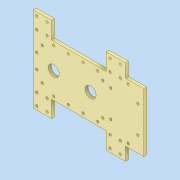
# Autodesk Inventor part: 130底盘5.0
Saved by Autodesk Inventor 2019 (Build 230136000, 136)
## iProperties
Created: 2020-11-07
Part Number: 130底盘5.0
Material: 尼龙 6/6
Document SubType Name: Modeling
Designer: Wang Hua
Density: 1.13 g/cm^3
Appearance: 尼龙 6
Author: Wang Hua
Autodesk Inventor part; units mm, degrees
ref_plane "YZ Plane" through (0, 0, 0) normal (1, 0, 0) x (0, 1, 0)
ref_plane "XZ Plane" through (0, 0, 0) normal (0, 1, 0) x (-1, 0, 0)
ref_plane "XY Plane" through (0, 0, 0) normal (0, 0, 1) x (1, 0, 0)
sketch "草图1" plane through (0, 0, 0) normal (0, 0, 1) x (1, 0, 0)
  line L0 (-136.9893, 0) -> (-136.9893, 58)
  line L1 (-136.9893, 58) -> (-111.9893, 58)
  line L2 (-111.9893, 58) -> (-111.9893, 35)
  line L3 (-111.9893, 35) -> (-37.7393, 35)
  line L4 (-37.7393, 35) -> (-37.7393, 58)
  line L5 (-37.7393, 58) -> (-11.2393, 58)
  line L6 (-167.1393, 0) -> (43.9107, 0) construction
  line L7 (-11.2393, 58) -> (-11.2393, 40)
  line L8 (-11.2393, 40) -> (13.7607, 40)
  line L9 (13.7607, 40) -> (13.7607, 0)
  circle A0 centre (-108.9469, 0) radius 7.5
  line L10 (-136.9893, 0) -> (-136.9893, -58)
  line L11 (-136.9893, -58) -> (-111.9893, -58)
  line L12 (-111.9893, -58) -> (-111.9893, -35)
  line L13 (-111.9893, -35) -> (-37.7393, -35)
  line L14 (-37.7393, -35) -> (-37.7393, -58)
  line L15 (-37.7393, -58) -> (-11.2393, -58)
  line L16 (-11.2393, -58) -> (-11.2393, -40)
  line L17 (-11.2393, -40) -> (13.7607, -40)
  line L18 (13.7607, -40) -> (13.7607, 0)
  circle A1 centre (-58.7806, 0) radius 7.5
  point P0 (0, 0)
  point P1 (-131.9893, 53)
  point P2 (-117.9898, 52.8821)
  point P3 (-131.9893, 37)
  point P4 (-117.9893, 36.8821)
  point P5 (-124.4893, 22.14)
  point P6 (-41.9893, 22.14)
  point P7 (-31.2393, 18.5)
  point P8 (5.7607, 18.5)
  point P9 (-108.9469, 30)
  point P10 (-88.9469, 30)
  point P11 (-68.9469, 30)
  point P12 (-48.9469, 30)
  point P13 (-131.9893, 10)
  point P14 (-131.9893, -53)
  point P15 (-117.9898, -52.8821)
  point P16 (-131.9893, -37)
  point P17 (-117.9893, -36.8821)
  point P18 (-124.4893, -22.14)
  point P19 (-41.9893, -22.14)
  point P20 (-31.2393, -18.5)
  point P21 (5.7607, -18.5)
  point P22 (-108.9469, -30)
  point P23 (-88.9469, -30)
  point P24 (-68.9469, -30)
  point P25 (-48.9469, -30)
  point P26 (-131.9893, -10)
  point P27 (-7.5117, 35)
  point P28 (-7.5117, -35)
  dimension "d0" = 58
  dimension "d1" = 25
  dimension "d2" = 26.5
  dimension "d4" = 35
  dimension "d6" = 40
  dimension "d7" = 14
  dimension "d8" = 16
  dimension "d9" = 5
  dimension "d10" = 5
  dimension "d11" = 14
  dimension "d12" = 16
  dimension "d13" = 5
  dimension "d14" = 25
  dimension "d15" = 82.5
  dimension "d16" = 22.14
  dimension "d17" = 15
  dimension "d18" = 37
  dimension "d19" = 8
  dimension "d20" = 18.5
  dimension "d21" = 18.5
  dimension "d22" = 5
  dimension "d23" = 5
  dimension "d24" = 5
  dimension "d25" = 5
  dimension "d26" = 20
  dimension "d27" = 20
  dimension "d28" = 20
  dimension "d29" = 10
  dimension "d30" = 15
  dimension "d41" = 5
  constraints: 36 end point, 22 symmetric about line, 8 point on line, 6 perpendicular, 2 centre point, 2 vertical
  measures "d0" distance of L0.start L0.end
  measures "d1" distance of L0.end L1.end
  measures "d2" distance of L4.end L5.end
  measures "d4" distance between parallel lines of L6 L3
  measures "d6" distance of L8.end L9.end
  measures "d7" distance of point (-117.99, 52.882) point (-131.989, 53)
  measures "d8" distance of point (-131.989, 37) point (-131.989, 53)
  measures "d9" distance from line of L1 point (-131.989, 53)
  measures "d10" distance from line of L0 point (-131.989, 53)
  measures "d11" horizontal distance of point (-117.989, 36.882) point (-131.989, 37)
  measures "d12" distance of point (-117.99, 52.882) point (-117.989, 36.882)
  measures "d13" distance from line of point (-131.989, 37) L0
  measures "d14" distance of L7.end L8.end
  measures "d15" distance of point (-41.989, 22.14) point (-124.489, 22.14)
  measures "d16" distance from line of L6 point (-124.489, 22.14)
  measures "d17" diameter of A0
  measures "d18" distance of point (5.761, 18.5) point (-31.239, 18.5)
  measures "d19" distance from line of L9 point (5.761, 18.5)
  measures "d20" distance from line of L6 point (-31.239, 18.5)
  measures "d21" distance from line of L6 point (5.761, 18.5)
  measures "d22" distance from line of L3 point (-108.947, 30)
  measures "d23" distance from line of L3 point (-88.947, 30)
  measures "d24" distance from line of L3 point (-68.947, 30)
  measures "d25" distance from line of L3 point (-48.947, 30)
  measures "d26" distance of point (-88.947, 30) point (-108.947, 30)
  measures "d27" distance of point (-68.947, 30) point (-88.947, 30)
  measures "d28" distance of point (-48.947, 30) point (-68.947, 30)
  measures "d29" distance from line of L6 point (-131.989, 10)
  measures "d30" diameter of A1
  measures "d41" distance from line of L8 point (-7.512, 35)
extrude "拉伸1" add sketch "草图1" along normal blind 4
hole "孔2" at (-131.9893, 53, 0) at (-117.9898, 52.8821, 0) at (-131.9893, 37, 0) at (-117.9893, 36.8821, 0) at (-124.4893, 22.14, 0) at (-41.9893, 22.14, 0) at (-31.2393, 18.5, 0) at (5.7607, 18.5, 0) at (-108.9469, 30, 0) at (-88.9469, 30, 0) at (-68.9469, 30, 0) at (-48.9469, 30, 0) at (-131.9893, 10, 0) at (-131.9893, -53, 0) at (-117.9898, -52.8821, 0) at (-117.9893, -36.8821, 0) at (-131.9893, -37, 0) at (-131.9893, -10, 0) at (-124.4893, -22.14, 0) at (-108.9469, -30, 0) at (-88.9469, -30, 0) at (-68.9469, -30, 0) at (-48.9469, -30, 0) at (5.7607, -18.5, 0) at (-31.2393, -18.5, 0) at (-41.9893, -22.14, 0) at (-7.5117, 35, 0) at (-7.5117, -35, 0) direction (0, 0, 1) diameter 3.2 end through all
sketch "草图2" plane through (0, 0, 4) normal (0, 0, 1) x (1, 0, 0)
  circle A0 centre (-7.5117, 35) radius 1.6 construction
  circle A1 centre (-31.2393, -18.5) radius 1.6 construction
  circle A2 centre (-48.9469, -30) radius 1.6 construction
  circle A3 centre (-88.9469, -30) radius 1.6 construction
  circle A4 centre (-124.4893, -22.14) radius 1.6 construction
  circle A5 centre (-131.9893, -37) radius 1.6 construction
  circle A6 centre (-117.9898, -52.8821) radius 1.6 construction
  circle A7 centre (-131.9893, 10) radius 1.6 construction
  circle A8 centre (-68.9469, 30) radius 1.6 construction
  circle A9 centre (-108.9469, 30) radius 1.6 construction
  circle A10 centre (-31.2393, 18.5) radius 1.6 construction
  circle A11 centre (-124.4893, 22.14) radius 1.6 construction
  circle A12 centre (-131.9893, 37) radius 1.6 construction
  circle A13 centre (-131.9893, 53) radius 1.6 construction
  circle A14 centre (-117.9898, 52.8821) radius 1.6 construction
  circle A15 centre (-117.9893, 36.8821) radius 1.6 construction
  circle A16 centre (-41.9893, 22.14) radius 1.6 construction
  circle A17 centre (5.7607, 18.5) radius 1.6 construction
  circle A18 centre (-88.9469, 30) radius 1.6 construction
  circle A19 centre (-48.9469, 30) radius 1.6 construction
  circle A20 centre (-131.9893, -53) radius 1.6 construction
  circle A21 centre (-117.9893, -36.8821) radius 1.6 construction
  circle A22 centre (-131.9893, -10) radius 1.6 construction
  circle A23 centre (-108.9469, -30) radius 1.6 construction
  circle A24 centre (-68.9469, -30) radius 1.6 construction
  circle A25 centre (5.7607, -18.5) radius 1.6 construction
  circle A26 centre (-41.9893, -22.14) radius 1.6 construction
  circle A27 centre (-7.5117, -35) radius 1.6 construction
  circle A28 centre (-58.7806, 0) radius 7.5 construction
  circle A29 centre (-108.9469, 0) radius 7.5 construction
  line L0 (-136.9893, 58) -> (-136.9893, -58) construction
  line L1 (-136.9893, -58) -> (-111.9893, -58) construction
  line L2 (-111.9893, -58) -> (-111.9893, -35) construction
  line L3 (-111.9893, -35) -> (-37.7393, -35) construction
  line L4 (-37.7393, -35) -> (-37.7393, -58) construction
  line L5 (-37.7393, -58) -> (-11.2393, -58) construction
  line L6 (-11.2393, -58) -> (-11.2393, -40) construction
  line L7 (-11.2393, -40) -> (13.7607, -40) construction
  line L8 (13.7607, -40) -> (13.7607, 40) construction
  line L9 (13.7607, 40) -> (-11.2393, 40) construction
  line L10 (-11.2393, 40) -> (-11.2393, 58) construction
  line L11 (-11.2393, 58) -> (-37.7393, 58) construction
  line L12 (-37.7393, 58) -> (-37.7393, 35) construction
  line L13 (-37.7393, 35) -> (-111.9893, 35) construction
  line L14 (-111.9893, 35) -> (-111.9893, 58) construction
  line L15 (-111.9893, 58) -> (-136.9893, 58) construction
  line L16 (0, 0) -> (-58.7806, 0) construction
  point P0 (-32.1393, 36.9745)
  point P1 (-18.1393, 36.9745)
  point P2 (-18.1393, 52.9745)
  point P3 (-32.1393, 52.9745)
  point P4 (-32.1393, -36.9745)
  point P5 (-18.1393, -36.9745)
  point P6 (-18.1393, -52.9745)
  point P7 (-32.1393, -52.9745)
  dimension "d49" = 16
  dimension "d50" = 14
  dimension "d51" = 14
  dimension "d52" = 16
  dimension "d53" = 5.6
  constraints: 4 symmetric about line, 2 end point, 1 horizontal
  measures "d49" distance of point (-32.139, 52.975) point (-32.139, 36.975)
  measures "d50" distance of point (-18.139, 36.975) point (-32.139, 36.975)
  measures "d51" distance of point (-32.139, 52.975) point (-18.139, 52.975)
  measures "d52" distance of point (-18.139, 36.975) point (-18.139, 52.975)
  measures "d53" distance from line of L12 point (-32.139, 52.975)
hole "孔3" at (-32.1393, 36.9745, 4) at (-18.1393, 36.9745, 4) at (-18.1393, 52.9745, 4) at (-32.1393, 52.9745, 4) at (-32.1393, -36.9745, 4) at (-18.1393, -36.9745, 4) at (-18.1393, -52.9745, 4) at (-32.1393, -52.9745, 4) direction (0, 0, -1) diameter 3.2 end through all
